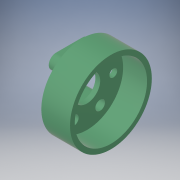
# Autodesk Inventor part: AS5047DEnclosureV2
Saved by Autodesk Inventor 2019.1 (Build 231200000, 200)
## iProperties
Created: 2018-06-30
Part Number: AS5047DEnclosureV2
Material: Generisch
Document SubType Name: Modeling
Designer: JochenAlt
Density: 1 g/cm^3
Appearance: Glatt - dunkelseegrün
Author: JochenAlt
Autodesk Inventor part; units mm, degrees
ref_plane "YZ Plane" through (0, 0, 0) normal (1, 0, 0) x (0, 1, 0)
ref_plane "XZ Plane" through (0, 0, 0) normal (0, 1, 0) x (-1, 0, 0)
ref_plane "XY Plane" through (0, 0, 0) normal (0, 0, 1) x (1, 0, 0)
ref_plane "Arbeitsebene1" through (0, 0, 0) normal (1, 0, 0) x (0, 0, -1)
sketch "Skizze1" plane through (0, 0, 0) normal (1, 0, 0) x (0, 0, -1)
  arc A0 (15.1, 0) -> (-15.1, 0) centre (0, 0) ccw
  circle A1 centre (0, 0) radius 5.5
  line L0 (-23.94, 0) -> (23.94, 0) construction
  line L1 (0, -23.94) -> (0, 23.94) construction
  line L2 (8.89, -5.5) -> (-8.89, -5.5) construction
  line L3 (-8.89, -5.5) -> (-8.89, 5.5) construction
  line L4 (-8.89, 5.5) -> (8.89, 5.5) construction
  line L5 (8.89, 5.5) -> (8.89, -5.5) construction
  circle A2 centre (8.89, 5.5) radius 1.2
  circle A3 centre (-8.89, 5.5) radius 1.2
  arc A4 (-15.1, 0) -> (14.6816, 3.5299) centre (0, 0) ccw
  arc A5 (4.4, 3.3) -> (-4.4, 3.3) centre (0, 0) ccw
  circle A6 centre (8.89, -5.5) radius 1.2
  circle A7 centre (-8.89, -5.5) radius 1.2
  line L6 (11.89, -5.5) -> (11.89, 5.5)
  line L7 (-5.89, -5.5) -> (-5.89, 5.5)
  line L8 (-11.89, -5.5) -> (-11.89, 5.5)
  arc A8 (-5.89, 5.5) -> (-11.89, 5.5) centre (-8.89, 5.5) ccw
  arc A9 (11.89, 5.5) -> (5.89, 5.5) centre (8.89, 5.5) ccw
  line L9 (5.89, -5.5) -> (5.89, 5.5)
  circle A10 centre (0, 0) radius 17.1
  circle A11 centre (-8.89, -5.5) radius 2
  circle A12 centre (8.89, -5.5) radius 2
  circle A13 centre (8.89, 5.5) radius 2
  circle A14 centre (-8.89, 5.5) radius 2
  circle A15 centre (0, 0) radius 11 construction
  circle A16 centre (0, 11) radius 1.6
  circle A17 centre (0, -11) radius 1.6
  arc A18 (-11.89, -5.5) -> (-5.89, -5.5) centre (-8.89, -5.5) ccw
  arc A19 (5.89, -5.5) -> (11.89, -5.5) centre (8.89, -5.5) ccw
  point P0 (0, 15.1)
  dimension "d2" = 11
  dimension "d19" = 11
  dimension "d20" = 17.78
  dimension "d22" = 2.4
  dimension "d29" = 15.1
  dimension "d30" = 5.5
  dimension "d38" = 3
  dimension "d44" = 2
  dimension "d51" = 4
  dimension "d52" = 22
  dimension "d53" = 3.2
  constraints: 20 centre point, 19 point on circle, 16 coincident, 16 end point, 8 equal radius, 8 tangent, 3 parallel, 2 point on line, 1 horizontal, 1 perpendicular, 3 other
  measures "d2" diameter of A1
  measures "d19" distance of L2.end L3.end
  measures "d20" distance of L3.end L4.end
  measures "d22" diameter of A2
  measures "d29" radius of A4
  measures "d30" radius of A5
  measures "d38" radius of A8
  measures "d44" radial gap between concentric circles of A10 A4
  measures "d51" diameter of A11
  measures "d52" diameter of A15
  measures "d53" diameter of A16
extrude "Extrusion7" add sketch "Skizze1" along normal blind 2 contours A4 A0 | A19 L9 A9 L6 | A18 L8 A8 L7 | A10
extrude "Extrusion3" add sketch "Skizze1" against normal blind 2.5 from surface at 0 contours A19 L9 A9 L6 | A18 L8 A8 L7
extrude "Extrusion4" add sketch "Skizze1" against normal blind 3 from surface at -2.5 contours A19 L9 A9 L6 | A18 L8 A8 L7 | A11 | A12 | A13 | A14
extrude "Extrusion8" add sketch "Skizze1" along normal blind 10 from surface at 2 contours A10
